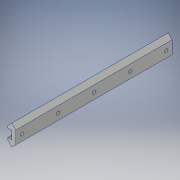
# Autodesk Inventor part: SC Path
Saved by Autodesk Inventor 2018.3 (Build 223284000, 284)
## iProperties
Created: 2020-02-15
Part Number: SC Path
Material: Aluminum 6061
Document SubType Name: Modeling
Designer: 22jungchan
Density: 2.7 g/cm^3
Appearance: Aluminum - Flat
Mass: 146.817 g
Surface Area: 197.478 cm^2
Volume: 54.3767 cm^3
Author: 22jungchan
Autodesk Inventor part; units mm, degrees
ref_plane "YZ Plane" through (0, 0, 0) normal (1, 0, 0) x (0, 1, 0)
sketch "Sketch1" plane through (0, 0, 0) normal (0, 0, 1) x (1, 0, 0)
  line L0 (0, 0) -> (12.7, 0)
  line L1 (12.7, 0) -> (12.7, -20.32)
  line L2 (12.7, -20.32) -> (0, -20.32)
  line L3 (0, -20.32) -> (0, 0)
  line L4 (0, 0) -> (6.35, 6.35)
  line L5 (12.7, -20.32) -> (6.35, -26.67)
  line L6 (6.35, -26.67) -> (0, -20.32)
  line L7 (6.35, 6.35) -> (12.7, 0)
  dimension "d0" = 90
  dimension "d1" = 90
  dimension "d2" = 33.02
  dimension "d3" = 12.7
  constraints: 16 end point, 2 equal length, 2 parallel, 1 horizontal, 1 perpendicular
  measures "d0" angle of L5 L6
  measures "d1" angle of L4 L7
  measures "d2" distance of L5.end L4.end
  measures "d3" distance between parallel lines of L1 L3
extrude "Extrusion1" add sketch "Sketch1" along normal blind 247.65
sketch "Sketch6" plane through (0, 0, 247.65) normal (0, 0, 1) x (1, 0, 0)
  line L0 (-5.8804, -3.81) -> (6.35, -3.81)
  line L1 (6.35, -3.81) -> (6.35, -16.51)
  line L2 (6.35, -16.51) -> (-5.8804, -16.51)
  line L3 (-5.8804, -16.51) -> (-5.8804, -3.81)
  line L4 (12.7, -20.32) -> (12.7, 0) projected
  line L5 (0, 0) -> (0, -20.32) projected
  point P0 (6.35, -10.16)
  point P1 (12.7, -10.16)
  dimension "d43" = 12.7
  dimension "d44" = 6.35
  constraints: 8 end point, 2 midpoint, 2 parallel, 1 horizontal, 1 horizontal alignment, 1 perpendicular
  measures "d43" distance of L2.end L0.start
  measures "d44" distance between parallel lines of L1 L5
extrude "Extrusion5" cut sketch "Sketch6" against normal through all
ref_plane "Work Plane1" through (6.35, -20.32, 0) normal (1, 0, 0) x (0, 0, -1)
ref_plane "Work Plane2" through (0, -10.16, 0) normal (0, 1, 0) x (-1, 0, 0)
sketch "Sketch2" plane through (12.7, -20.32, 0) normal (1, 0, 0) x (0, 0, -1)
  line L0 (-247.65, 0) -> (-247.65, 20.32) projected
  line L1 (0, 20.32) -> (-247.65, 20.32) projected
  line L2 (0, 20.32) -> (0, 0) projected
  line L3 (0, 0) -> (-247.65, 0) projected
  circle A0 centre (-238.125, 10.16) radius 4.7625
  circle A1 centre (-9.525, 10.16) radius 4.7625
  line L4 (-233.3625, 16.7388) -> (-233.3625, 5.4122)
  line L5 (-14.2875, 15.6909) -> (-14.2875, 3.5669)
  point P0 (0, 10.16)
  point P1 (-180.975, 10.16)
  point P2 (-66.675, 10.16)
  point P3 (-123.825, 10.16)
  dimension "d28" = 9.525
  dimension "d47" = 9.525
  dimension "d48" = 57.15
  dimension "d49" = 57.15
  dimension "d51" = 9.525
  dimension "d52" = 219.075
  dimension "d56" = 57.15
  dimension "d59" = 228.6
  dimension "d60" = 57.15
  constraints: 5 horizontal alignment, 4 end point, 2 centre point, 2 coincident, 2 tangent, 1 equal radius, 1 midpoint, 1 parallel, 1 vertical
  measures "d28" distance from line of L2 point (-9.525, 10.16)
  measures "d47" distance from line of point (-238.125, 10.16) L0
  measures "d48" distance of point (-180.975, 10.16) point (-238.125, 10.16)
  measures "d49" distance of point (-9.525, 10.16) point (-66.675, 10.16)
  measures "d51" diameter of A0
  measures "d52" distance between parallel lines of L5 L4
  measures "d56" distance of point (-66.675, 10.16) point (-123.825, 10.16)
  measures "d59" distance of point (-9.525, 10.16) point (-238.125, 10.16)
  measures "d60" distance of point (-123.825, 10.16) point (-180.975, 10.16)
hole "Hole2" at (12.7, -10.16, 9.525) at (12.7, -10.16, 180.975) at (12.7, -10.16, 66.675) at (12.7, -10.16, 238.125) at (12.7, -10.16, 123.825) direction (-1, 0, 0) diameter 5.1054 end through all clearance for "Flat Head Machine Screw (82)" size "#10" standard "Ansi Unified Screw Threads"
body "Solid1"
